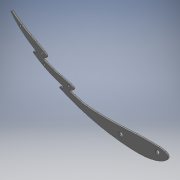
# Autodesk Inventor part: bracket2
Saved by Autodesk Inventor 2018 (Build 220112000, 112)
## iProperties
Created: 2018-03-05
Part Number: bracket2
Material: 木材 (オーク)
Document SubType Name: Modeling
Designer: ku_sk
Density: 0.76 g/cm^3
Appearance: ホワイト オーク材 - ナチュラル 標準の光沢
Author: ku_sk
Autodesk Inventor part; units mm, degrees
ref_plane "YZ Plane" through (0, 0, 0) normal (1, 0, 0) x (0, 1, 0)
ref_plane "XZ Plane" through (0, 0, 0) normal (0, 1, 0) x (-1, 0, 0)
ref_plane "XY Plane" through (0, 0, 0) normal (0, 0, 1) x (1, 0, 0)
sketch "スケッチ2" plane through (0, 0, 0) normal (0, 1, 0) x (-1, 0, 0)
  circle A0 centre (366.8992, 83.5559) radius 3 projected
  circle A1 centre (432.0925, 120.7557) radius 3 projected
  arc A2 (460.0993, 143.4366) -> (457.2735, 146.2345) centre (458.5344, 144.682) ccw projected
  arc A3 (400.439, 89.2207) -> (460.0993, 143.4366) centre (263.302, 300.0629) ccw projected
  arc A4 (391.277, 83.6402) -> (400.439, 89.2207) centre (301.619, 241.1522) ccw projected
  arc A5 (372.7132, 76.1699) -> (391.277, 83.6402) centre (354.4726, 148.2986) ccw projected
  arc A6 (360.1081, 74.8804) -> (372.7132, 76.1699) centre (362.0183, 118.4608) ccw projected
  arc A7 (355.7086, 75.8282) -> (360.1081, 74.8804) centre (360.696, 88.2936) ccw projected
  arc A8 (354.3762, 83.2451) -> (355.7086, 75.8282) centre (357.3588, 79.9528) ccw projected
  arc A9 (361.0987, 88.3442) -> (354.3762, 83.2451) centre (386.9085, 47.3355) ccw projected
  arc A10 (385.4553, 102.095) -> (361.0987, 88.3442) centre (517.0615, -159.4623) ccw projected
  arc A11 (385.4553, 102.095) -> (400.8032, 109.8486) centre (-2010.0977, 4863.0707) ccw projected
  arc A12 (400.8032, 109.8486) -> (428.5996, 125.6368) centre (247.4107, 412.2703) ccw projected
  arc A13 (428.5996, 125.6368) -> (457.2735, 146.2345) centre (269.2327, 377.7487) ccw projected
  circle A14 centre (287.1934, 37.1564) radius 3 projected
  circle A15 centre (359.7933, 56.2153) radius 3 projected
  arc A16 (392.7161, 70.8747) -> (390.7107, 74.3087) centre (391.5269, 72.4828) ccw projected
  arc A17 (321.0565, 33.9474) -> (392.7161, 70.8747) centre (243.1623, 273.099) ccw projected
  arc A18 (310.7624, 30.9284) -> (321.0565, 33.9474) centre (264.9264, 206.2785) ccw projected
  arc A19 (290.8977, 28.5173) -> (310.7624, 30.9284) centre (291.9468, 102.9093) ccw projected
  arc A20 (278.3883, 30.5342) -> (290.8977, 28.5173) centre (291.5128, 72.1352) ccw projected
  arc A21 (274.384, 32.5883) -> (278.3883, 30.5342) centre (282.4278, 43.3382) ccw projected
  arc A22 (275.0166, 40.0974) -> (274.384, 32.5883) centre (277.0456, 36.1453) ccw projected
  arc A23 (282.8299, 43.2828) -> (275.0166, 40.0974) centre (297.1464, -3.0086) ccw projected
  arc A24 (309.9154, 50.2611) -> (282.8299, 43.2828) centre (369.3413, -236.446) ccw projected
  arc A25 (309.9154, 50.2611) -> (326.7472, 53.7782) centre (-771.7798, 5269.0252) ccw projected
  arc A26 (326.7472, 53.7782) -> (357.6827, 61.8342) centre (256.8539, 385.5961) ccw projected
  arc A27 (357.6827, 61.8342) -> (390.7107, 74.3087) centre (268.9975, 346.6028) ccw projected
  circle A28 centre (20.0666, -1.5588) radius 5 projected
  circle A29 centre (130.4331, -10.1322) radius 5 projected
  arc A30 (313.248, 18.4984) -> (312.0524, 22.2894) centre (312.4376, 20.3268) ccw projected
  arc A31 (100.6618, -32.4332) -> (313.248, 18.4984) centre (68.6386, 570.3585) ccw projected
  arc A32 (74.9225, -33.0376) -> (100.6618, -32.4332) centre (77.5861, 401.9345) ccw projected
  arc A33 (27.374, -26.2879) -> (74.9225, -33.0376) centre (76.0159, 145.5175) ccw projected
  arc A34 (-0.3728, -13.8419) -> (27.374, -26.2879) centre (55.8939, 74.446) ccw projected
  arc A35 (-8.3795, -6.5926) -> (-0.3728, -13.8419) centre (16.9451, 13.3315) ccw projected
  arc A36 (-2.2486, 10.4222) -> (-8.3795, -6.5926) centre (0, 0) ccw projected
  arc A37 (17.8428, 12.9532) -> (-2.2486, 10.4222) centre (22.277, -103.2534) ccw projected
  arc A38 (84.9679, 12.306) -> (17.8428, 12.9532) centre (44.6377, -689.2581) ccw projected
  arc A39 (84.9679, 12.306) -> (126.1724, 10.004) centre (819.0754, 12782.4716) ccw projected
  arc A40 (126.1724, 10.004) -> (202.8919, 9.4636) centre (170.258, 822.6468) ccw projected
  arc A41 (202.8919, 9.4636) -> (312.0524, 22.2894) centre (174.1884, 724.7085) ccw projected
  line L0 (400.439, 89.2207) -> (374.6007, 72.4148)
  line L1 (374.6007, 72.4148) -> (391.2826, 74.4678)
  line L2 (355.7086, 75.8282) -> (369.1755, 70.4401)
  line L3 (369.1755, 70.4401) -> (326.7472, 53.7782)
  line L4 (321.0565, 33.9474) -> (289.8884, 23.7957)
  line L5 (289.8884, 23.7957) -> (312.5672, 22.3226)
  line L6 (278.3883, 30.5342) -> (291.6044, 26.3646)
  line L7 (291.6044, 26.3646) -> (243.2783, 12.2299)
  point P0 (0, 0)
  constraints: 16 end point, 6 tangent, 3 point on circle
extrude "押し出し2" add sketch "スケッチ2" along normal blind 4
fillet "フィレット2" radius 3 4 edges at (-369.1755, 2, 70.4401) (-291.6044, 2, 26.3646) (-374.6007, 2, 72.4148) (-289.8884, 2, 23.7957)
fillet "フィレット2" radius 100 2 edges at (-326.7472, 2, 53.7782) (-243.2783, 2, 12.2299)
sketch "スケッチ3" plane through (0, 0, 0) normal (0, -1, 0) x (1, 0, 0)
  circle A0 centre (-20.0666, -1.5588) radius 6
  circle A1 centre (-130.4331, -10.1322) radius 6
  circle A2 centre (-130.4331, -10.1322) radius 5 projected
  circle A3 centre (-20.0666, -1.5588) radius 5 projected
  point P0 (0, 0)
  dimension "d10" = 12
  dimension "d11" = 12
  constraints: 2 centre point, 2 concentric
  measures "d10" diameter of A1
  measures "d11" diameter of A0
extrude "押し出し3" cut sketch "スケッチ3" against normal through all
equation "\"d11\" = d10"
